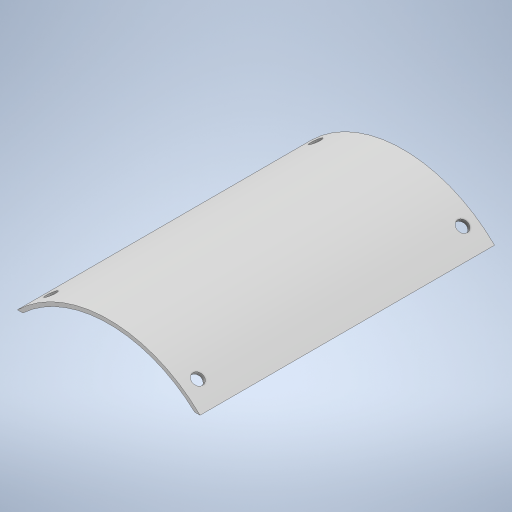
# Autodesk Inventor part: Electronics Door
Saved by Autodesk Inventor 2024 (Build 280153000, 153)
## iProperties
Created: 2024-04-23
Part Number: Electronics Door
Material: Generic
Document SubType Name: Modeling
Designer: auror
Density: 1 g/cm^3
Appearance: Default
Author: auror
Autodesk Inventor part; units mm, degrees
ref_plane "YZ Plane" through (0, 0, 0) normal (1, 0, 0) x (0, 1, 0)
ref_plane "XZ Plane" through (0, 0, 0) normal (0, 1, 0) x (-1, 0, 0)
ref_plane "XY Plane" through (0, 0, 0) normal (0, 0, 1) x (1, 0, 0)
sketch "Sketch8" plane through (0, 0, 0) normal (0, 0, 1) x (1, 0, 0)
  arc A0 (23.0521, 24.992) -> (-23.0521, 24.992) centre (0, 0) ccw
  arc A1 (24.495, 24.9999) -> (-24.495, 24.9999) centre (0, 0) ccw
  line L0 (-23.0521, 24.992) -> (-24.495, 24.9999)
  line L1 (-23.9428, 24.1705) -> (-22.1865, 25.7904) construction
  line L2 (22.2643, 25.7187) -> (23.852, 24.2542) construction
  line L3 (23.0521, 24.992) -> (24.495, 24.9999)
  line L4 (-24.495, 24.9999) -> (24.495, 24.9999) construction
  dimension "d88" = 34
  dimension "d89" = 35
  dimension "d90" = 0
  dimension "d91" = 137
  dimension "d92" = 0
  dimension "d93" = 137
  dimension "d98" = 48.99
  constraints: 10 end point, 4 point on circle, 2 centre point, 2 coincident, 2 tangent, 1 horizontal
  measures "d88" radius of A0
  measures "d89" radius of A1
  measures "d90" distance from line of L0.start L1
  measures "d91" angle of L0 L1
  measures "d92" distance from line of L3.start L2
  measures "d93" angle of L3 L2
  measures "d98" distance of L0.end L3.end
extrude "Extrusion5" add sketch "Sketch8" along normal blind 79
sketch "Sketch19" plane through (0, 0, 79) normal (0, 0, 1) x (1, 0, 0)
  line L0 (-24.495, 24.9999) -> (-23.0521, 24.992) construction
  line L1 (-22.2755, 25.021) -> (-7.4699, 32.6566) construction
  arc A0 (22.2755, 25.021) -> (-22.2755, 25.021) centre (0, 0) ccw construction
  dimension "d162" = 32.448
  constraints: 2 end point, 1 point on circle, 1 other
  measures "d162" distance from line of point (0, 0) L1
sketch "Sketch22" plane through (0, 0, 79) normal (0, 0, 1) x (1, 0, 0)
  line L0 (0, 0) -> (23.3944, 25.3632) construction
  line L1 (0, 0) -> (30.8624, 21.8617) construction
  arc A0 (23.0521, 24.992) -> (-23.0521, 24.992) centre (0, 0) ccw construction
  arc A1 (29.7973, 16.3744) -> (23.0521, 24.992) centre (0, 0) ccw construction
  line L2 (27.7445, 19.6531) -> (8.8852, 32.8185) construction
  point P0 (19.0454, 25.7258)
  dimension "d175" = 12
  dimension "d176" = 23
  dimension "d177" = 0
  dimension "d178" = 10.609
  constraints: 6 end point, 4 point on circle, 2 point on line, 1 centre point, 1 coincident
  measures "d175" angle of L0 L1
  measures "d176" distance of L2.start L2.end
  measures "d177" distance from line of A0.start L0
  measures "d178" distance of L2.start point (19.045, 25.726)
sketch "Sketch23" plane through (0, 0, 0) normal (0, 0, -1) x (-1, 0, 0)
  arc A0 (23.0521, 24.992) -> (-23.0521, 24.992) centre (0, 0) ccw projected
  line L0 (0, 0) -> (-23.0521, 24.992) construction
  line L1 (0, 0) -> (-30.5798, 21.6616) construction
  arc A1 (-23.0521, 24.992) -> (-29.6271, 16.6805) centre (0, 0) ccw construction
  line L2 (-27.7445, 19.6531) -> (-8.8852, 32.8185) construction
  dimension "d179" = 12
  dimension "d180" = 23
  constraints: 6 end point, 4 point on circle, 1 centre point, 1 coincident, 1 point on line
  measures "d179" angle of L0 L1
  measures "d180" distance of L2.start L2.end
ref_plane "Work Plane12" through (27.7445, 19.6531, 79) normal (-0.5724082, -0.8199688, 0) x (-0.8199688, 0.5724082, 0)
sketch "Sketch24" plane through (27.7445, 19.6531, 79) normal (-0.5724082, -0.8199688, 0) x (-0.8199688, 0.5724082, 0)
  line L0 (6.9037, 79) -> (6.9037, 0) projected
  line L1 (44.7076, 0) -> (6.9037, 0) projected
  line L2 (44.7076, 79) -> (6.9037, 79) projected
  point P0 (11.5, 79)
  point P1 (11.9037, 75.2)
  point P2 (11.9037, 4.2)
  dimension "d181" = 5
  dimension "d182" = 4.2
  dimension "d183" = 3.8
  dimension "d184" = 5
  measures "d181" distance from line of L0 point (11.904, 4.2)
  measures "d182" distance from line of point (11.904, 4.2) L1
  measures "d183" distance from line of L2 point (11.904, 75.2)
  measures "d184" distance from line of L0 point (11.904, 75.2)
hole "Hole11" at (17.9838, 26.4669, 3.8) at (17.9838, 26.4669, 74.8) direction (0.5724082, 0.8199688, 0) diameter 3.1 end through all
ref_plane "Work Plane13" through (0, 24.8664, 0) normal (-1, 0, 0) x (0, 0, -1)
mirror "Mirror2" about plane through (0, 24.8664, 0) normal (-1, 0, 0) of "Hole11"
body "Solid2"
